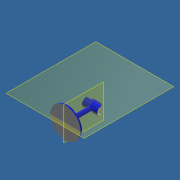
# Autodesk Inventor part: Feet
Saved by Autodesk Inventor 2018 (Build 220112000, 112)
## iProperties
Created: 2022-02-21
Part Number: Feet
Material: Generic
Document SubType Name: Modeling
Designer: Nathann
Density: 1 g/cm^3
Appearance: Default
Author: Nathann
Autodesk Inventor part; units mm, degrees
ref_plane "YZ Plane" through (0, 0, 0) normal (1, 0, 0) x (0, 1, 0)
ref_plane "XZ Plane" through (0, 0, 0) normal (0, 1, 0) x (-1, 0, 0)
ref_plane "XY Plane" through (0, 0, 0) normal (0, 0, 1) x (1, 0, 0)
sketch "Sketch1" plane through (0, 0, 0) normal (0, 1, 0) x (-1, 0, 0)
  circle A0 centre (0, 0) radius 100
  dimension "d0" = 200
  constraints: 1 centre point, 1 coincident
  measures "d0" diameter of A0
extrude "Extrusion1" add sketch "Sketch1" along normal blind 10
sketch "Sketch2" plane through (0, 10, 0) normal (0, 1, 0) x (1, 0, 0)
  circle A0 centre (0, 0) radius 15
  dimension "d5" = 30
  constraints: 1 centre point, 1 coincident
  measures "d5" diameter of A0
extrude "Extrusion2" add sketch "Sketch2" along normal blind 150
fillet "Fillet1" radius 20 1 edges at (-15, 10, 0)
sketch "Sketch3" plane through (0, 0, 0) normal (1, 0, 0) x (0, 1, 0)
  circle A0 centre (190, 0) radius 30
  line L0 (160, -15) -> (160, 15) projected
  circle A1 centre (190, 0) radius 25
  point P0 (0, 0)
  dimension "d7" = 50
  dimension "d8" = 60
  constraints: 2 centre point, 1 coincident, 1 tangent
  measures "d7" diameter of A1
  measures "d8" diameter of A0
extrude "Extrusion3" add sketch "Sketch3" along normal mid plane 40
sketch "Sketch5" plane through (20, 190, 0) normal (1, 0, 0) x (0, 0, -1)
  circle A0 centre (0, 0) radius 25 projected
  circle A1 centre (0, 0) radius 30 projected
  line L0 (-30, 0) -> (30, 0)
  circle A2 centre (0, 0) radius 30 projected
  arc A3 (-30, 0) -> (30, 0) centre (0, 0) ccw
  arc A4 (-25, 0) -> (25, 0) centre (0, 0) ccw
  point P0 (0, -190)
  constraints: 5 point on circle, 2 centre point, 2 coincident, 2 end point, 2 point on line, 1 horizontal, 1 horizontal alignment, 1 other
extrude "Extrusion5" add sketch "Sketch5" along normal blind 30 contours L0 A1 A0 picked at (27.8006, -4.3875)
ref_plane "Work Plane1" through (28.4663, -4.1462, 0) normal (0, 0, 1) x (1, 0, 0)
sketch "Sketch7" plane through (28.4663, -4.1462, 0) normal (0, 0, 1) x (1, 0, 0)
  circle A0 centre (16.5337, 191.1462) radius 1
  circle A1 centre (11.5337, 191.1462) radius 1
  line L0 (21.5337, 194.1462) -> (21.5337, 169.1462) projected
  line L1 (-8.4663, 194.1462) -> (21.5337, 194.1462) projected
  point P0 (-28.4663, 4.1462)
  dimension "d16" = 2
  dimension "d17" = 2
  dimension "d18" = 5
  dimension "d19" = 5
  dimension "d20" = 3
  dimension "d21" = 3
  constraints: 2 centre point
  measures "d16" diameter of A0
  measures "d17" diameter of A1
  measures "d18" distance from line of L0 A0.centre
  measures "d19" distance of A0.centre A1.centre
  measures "d20" distance from line of L1 A0.centre
  measures "d21" distance from line of L1 A1.centre
extrude "Extrusion6" cut sketch "Sketch7" along normal through all both and the other way through all
ref_plane "Work Plane2" through (0, 0, 0) normal (1, 0, 0) x (0, 0, -1)
mirror "Mirror1" about plane through (0, 0, 0) normal (1, 0, 0) of "Extrusion6", "Extrusion5"
sketch "Sketch8" plane through (-50, 190, 0) normal (-1, 0, 0) x (0, 0, 1)
  arc A0 (-25, 0) -> (25, 0) centre (0, 0) ccw projected
  line L0 (-25, 0) -> (-30, 0)
  line L1 (-30, 0) -> (-30, -27.8737)
  line L2 (-30, -27.8737) -> (-25, -27.8737)
  line L3 (-25, -27.8737) -> (-25, 0)
  line L4 (25, 0) -> (30, 0) projected
  line L5 (30, 0) -> (25, 0)
  line L6 (25, 0) -> (25, -27.8737)
  line L7 (25, -27.8737) -> (30, -27.8737)
  line L8 (30, -27.8737) -> (30, 0)
  point P0 (0, -190)
  constraints: 16 end point, 4 parallel, 2 horizontal, 2 perpendicular
extrude "Extrusion7" add sketch "Sketch8" along normal blind 5
sketch "Sketch9" plane through (-50, 162.1263, 30) normal (0, 0, 1) x (1, 0, 0)
  circle A0 centre (-3, 2) radius 1
  line L0 (0, 0) -> (-5, 0) projected
  line L1 (-5, 0) -> (-5, 27.8737) projected
  line L2 (-4, 2) -> (-4, 4.3193)
  line L3 (-2, 2) -> (-2, 4.3193)
  line L4 (-2, 4.3193) -> (0, 4.3193)
  line L5 (0, 11.2906) -> (0, 0) projected
  line L6 (0, 6.6143) -> (-2.9832, 6.6143)
  line L7 (-4, 5.6453) -> (-4, 4.3193)
  arc A1 (-2.9832, 6.6143) -> (-4, 5.6453) centre (-2.9832, 5.5963) ccw
  line L8 (0, 4.3193) -> (0, 6.6143)
  point P0 (50, -162.1263)
  dimension "d26" = 2
  dimension "d27" = 2
  dimension "d28" = 2
  constraints: 12 end point, 4 point on circle, 3 perpendicular, 2 centre point, 2 point on line, 2 vertical, 1 horizontal, 1 tangent
  measures "d26" diameter of A0
  measures "d27" distance from line of L0 A0.centre
  measures "d28" distance from line of L1 A0.centre
extrude "Extrusion8" cut sketch "Sketch9" against normal through all
body "Solid1"
